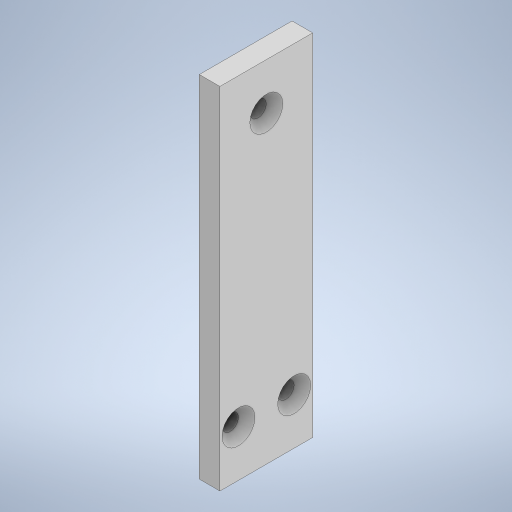
# Autodesk Inventor part: Sujetador prensa Trigger
Saved by Autodesk Inventor 2024.2 (Build 282272000, 272)
## iProperties
Created: 2026-07-03
Part Number: Sujetador prensa Trigger
Material: Generic
Document SubType Name: Modeling
Designer: ja.restrepo1
Density: 1 g/cm^3
Appearance: Default
Author: ja.restrepo1
Autodesk Inventor part; units mm, degrees
ref_plane "YZ Plane" through (0, 0, 0) normal (1, 0, 0) x (0, 1, 0)
ref_plane "XZ Plane" through (0, 0, 0) normal (0, 1, 0) x (-1, 0, 0)
ref_plane "XY Plane" through (0, 0, 0) normal (0, 0, 1) x (1, 0, 0)
sketch "Sketch1" plane through (0, 0, 0) normal (1, 0, 0) x (0, 1, 0)
  line L0 (85, 22.5) -> (-85, 22.5)
  line L1 (-85, 22.5) -> (-85, -22.5)
  line L2 (-85, -22.5) -> (85, -22.5)
  line L3 (85, -22.5) -> (85, 22.5)
  point P0 (0, 0)
  point P1 (85, 0)
  point P2 (0, 22.5)
  dimension "d0" = 170
  dimension "d1" = 45
  constraints: 8 end point, 2 midpoint, 2 parallel, 1 horizontal, 1 horizontal alignment, 1 perpendicular, 1 vertical alignment
  measures "d0" distance of L2.end L1.end
  measures "d1" distance of L1.end L0.end
extrude "Extrusion1" add sketch "Sketch1" along normal mid plane 10
sketch "Sketch2" plane through (5, 0, 0) normal (1, 0, 0) x (0, 0, -1)
  line L0 (-13.5, -62.5) -> (13.5, -62.5) construction
  line L1 (-22.5, -85) -> (22.5, -85) construction
  point P0 (0, 0)
  point P1 (0, -62.5)
  dimension "d4" = 27
  dimension "d5" = 22.5
  constraints: 2 end point, 1 horizontal, 1 midpoint, 1 vertical alignment
  measures "d4" distance of L0.start L0.end
  measures "d5" distance from line of L0.end L1
hole "BCA M8" at (5, -62.5, 13.5) at (5, -62.5, -13.5) direction (-1, 0, 0) diameter 8 end through all countersink diameter 16 countersink angle 90
sketch "Sketch3" plane through (5, 0, 0) normal (1, 0, 0) x (0, 0, -1)
  line L0 (22.5, 85) -> (-22.5, 85) projected
  point P0 (0, 0)
  point P1 (0, 62.5)
  dimension "d13" = 22.5
  constraints: 1 vertical alignment
  measures "d13" distance from line of L0 point (0, 62.5)
hole "Hole2" at (5, 62.5, 0) direction (-1, 0, 0) diameter 8 end through all countersink diameter 16 countersink angle 90
body "Solid1"
